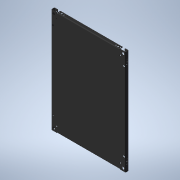
# Autodesk Inventor part: 8617.540_P1
Saved by Autodesk Inventor 2021 (Build 250183000, 183)
## iProperties
Created: 2026-08-04
Part Number: 8617.540_P1
Material: Generic
Catalog Web Link: www.3dfindit.com
Description: VX Teilmontageplatte - P1-VX Teilmontageplatte - P1
Vendor: RITTAL
Document SubType Name: Modeling
Designer: psAdmin
Manufacturer: RITTAL
Mass: 1032.29 g
Surface Area: 8360.76 cm^2
Volume: 1032.29 cm^3
Density: 1 g/cm^3
Appearance: PSOLRGB-176-176-176
Category: PARTsolutions
Company: RITTAL
Title: 8617.540_P1
Author: Cadenas PARTsolutions
Comments: VX Teilmontageplatte - P1
PSOL_IDENT_0: {$CADENAS_DATA/23d-libs/rittal/sys_zub/innenausbau/montageplatten/parts/teilmontageplatten_m51_p1.pr
PSOL_IDENT_1: j},181 {VTYP=3D},{NB=8617.540_P1},{LINA=8617.540_P1},{NN=VX Teilmontageplatte - P1},{DATE=16.02.2026
PSOL_IDENT_2: 20:13:30},{GEOMDATE=20.05.2025 11:57:00},{VERSION=},{LINEID=40},{WBVAR=},{WBNUMERIC=}  {NB=8617.540
PSOL_IDENT_3: _P1},{LINA=8617.540_P1},{KT=DUMMY},{BEST=8617.540},{INFO=PDF Katalog},{BEZ1=VX Teilmontageplatte},{B
PSOL_IDENT_4: EZ2=für neues Großschranksystem},{B=600},{BB=499},{H=800},{HH=699},{SB=600},{SH=800},{AB=600 x 800},
PSOL_IDENT_5: {VE=1},{VERS=4},{INFOPAGE=hb35_s707},{INFOPATH=hb35_s707_en.pdf},{CNSECLASS51=27-18-92-31},{CNSECLAS
PSOL_IDENT_6: S70=27-40-92-16},{CNSECLASS80=27-40-92-16},{CNSETIM40=EC000213},{BEZ3=},{DETAIL=1},{ADDGEO=1},{GEW=9
PSOL_IDENT_7: ,22},{CNSETIM80=EC000213},{CNSETIM90=EC000213},{CNSECLASS60=27-40-92-16},{UNSPSC=31-26-15-02}
NB: 8617.540_P1
NN: VX Teilmontageplatte - P1
NT: VX Teilmontageplatte - P1
NBSYN: $BEST._P1
LINA: 8617.540_P1
CATALOG: Rittal
BEST: 8617.540
INFO: PDF Katalog
BEZ1: VX Teilmontageplatte
BB: 499
HH: 699
SB: 600
SH: 800
CNSECLASS70: 27-40-92-16
CNSECLASS80: 27-40-92-16
GEW: 9,22
CNSETIM80: EC000213
CNSETIM90: EC000213
CNSECLASS60: 27-40-92-16
UNSPSC: 31-26-15-02
SUPPLIER: RITTAL
ARTICLENO: 8617.540_P1
BOMINFO: 8617.540_P1
CREATOR: CADENAS GmbH
Autodesk Inventor part; units mm, degrees
ref_plane "YZ Plane" through (0, 0, 0) normal (1, 0, 0) x (0, 1, 0)
ref_plane "XZ Plane" through (0, 0, 0) normal (0, 1, 0) x (-1, 0, 0)
ref_plane "XY Plane" through (0, 0, 0) normal (0, 0, 1) x (1, 0, 0)
sketch "Sketch_1" plane through (0, 0, 22) normal (0, 0, 1) x (1, 0, 0)
  line L0 (-244.5, 349.5) -> (-244.5, -349.5)
  line L1 (-244.5, -349.5) -> (-211.75, -349.5)
  line L2 (-211.75, -349.5) -> (-211.75, -344.5)
  arc A0 (-209.75, -344.5) -> (-211.75, -344.5) centre (-210.75, -344.5) ccw
  line L3 (-209.75, -344.5) -> (209.75, -344.5)
  arc A1 (211.75, -344.5) -> (209.75, -344.5) centre (210.75, -344.5) ccw
  line L4 (211.75, -344.5) -> (211.75, -349.5)
  line L5 (211.75, -349.5) -> (244.5, -349.5)
  line L6 (244.5, -349.5) -> (244.5, 349.5)
  line L7 (244.5, 349.5) -> (211.75, 349.5)
  line L8 (211.75, 349.5) -> (211.75, 344.5)
  arc A2 (209.75, 344.5) -> (211.75, 344.5) centre (210.75, 344.5) ccw
  line L9 (209.75, 344.5) -> (-209.75, 344.5)
  arc A3 (-211.75, 344.5) -> (-209.75, 344.5) centre (-210.75, 344.5) ccw
  line L10 (-211.75, 344.5) -> (-211.75, 349.5)
  line L11 (-211.75, 349.5) -> (-244.5, 349.5)
  circle A4 centre (237.5, 262.5) radius 6.25
  circle A5 centre (237.5, -262.5) radius 6.25
  circle A6 centre (232.5, 332.5) radius 8
  circle A7 centre (232.5, -332.5) radius 8
  circle A8 centre (213, 313) radius 4.5
  circle A9 centre (213, -313) radius 4.5
  circle A10 centre (-213, 313) radius 4.5
  circle A11 centre (-213, -313) radius 4.5
  circle A12 centre (-232.5, 332.5) radius 8
  circle A13 centre (-232.5, -332.5) radius 8
  circle A14 centre (-237.5, 262.5) radius 6.25
  circle A15 centre (-237.5, -262.5) radius 6.25
  constraints: 24 end point, 16 centre point, 8 point on circle
extrude "Extrusion1" add sketch "Sketch_1" against normal blind 2.5
sketch "Sketch_2" plane through (0, 0, 0) normal (0, 1, 0) x (1, 0, 0)
  line L0 (244.5, -19.5) -> (244.5, -22)
  arc A0 (244.5, -22) -> (249.5, -17) centre (244.5, -17) ccw
  line L1 (249.5, -17) -> (247, -17)
  arc A1 (244.5, -19.5) -> (247, -17) centre (244.5, -17) ccw
  constraints: 4 end point, 4 point on circle, 2 centre point
extrude "Extrusion2" add sketch "Sketch_2" along normal mid plane 699
sketch "Sketch_3" plane through (0, 0, 0) normal (0, 1, 0) x (1, 0, 0)
  arc A0 (-249.5, -17) -> (-244.5, -22) centre (-244.5, -17) ccw
  line L0 (-244.5, -22) -> (-244.5, -19.5)
  arc A1 (-247, -17) -> (-244.5, -19.5) centre (-244.5, -17) ccw
  line L1 (-247, -17) -> (-249.5, -17)
  constraints: 4 end point, 4 point on circle, 2 centre point
extrude "Extrusion3" add sketch "Sketch_3" along normal mid plane 699
sketch "Sketch_4" plane through (249.5, 0, 0) normal (1, 0, 0) x (0, 0, -1)
  line L0 (-17, 349.5) -> (-17, -349.5)
  line L1 (-17, -349.5) -> (-5, -349.5)
  line L2 (-5, -349.5) -> (-5, 349.5)
  line L3 (-5, 349.5) -> (-17, 349.5)
  circle A0 centre (-11, 304.5) radius 3.5
  circle A1 centre (-11, 274.5) radius 3.5
  circle A2 centre (-11, -304.5) radius 3.5
  circle A3 centre (-11, -274.5) radius 3.5
  circle A4 centre (-11, 289.5) radius 5.5
  circle A5 centre (-11, -289.5) radius 5.5
  constraints: 8 end point, 6 centre point
extrude "Extrusion4" add sketch "Sketch_4" against normal blind 2.5
sketch "Sketch_5" plane through (-249.5, 0, 0) normal (1, 0, 0) x (0, 0, -1)
  line L0 (-17, 349.5) -> (-17, -349.5)
  line L1 (-17, -349.5) -> (-5, -349.5)
  line L2 (-5, -349.5) -> (-5, 349.5)
  line L3 (-5, 349.5) -> (-17, 349.5)
  circle A0 centre (-11, 304.5) radius 3.5
  circle A1 centre (-11, 274.5) radius 3.5
  circle A2 centre (-11, -304.5) radius 3.5
  circle A3 centre (-11, -274.5) radius 3.5
  circle A4 centre (-11, 289.5) radius 5.5
  circle A5 centre (-11, -289.5) radius 5.5
  constraints: 8 end point, 6 centre point
extrude "Extrusion5" add sketch "Sketch_5" along normal blind 2.5
sketch "Sketch_6" plane through (0, 0, 0) normal (0, 1, 0) x (1, 0, 0)
  arc A0 (247, -5) -> (244.5, -2.5) centre (244.5, -5) ccw
  line L0 (247, -5) -> (249.5, -5)
  arc A1 (249.5, -5) -> (244.5, 0) centre (244.5, -5) ccw
  line L1 (244.5, 0) -> (244.5, -2.5)
  constraints: 4 end point, 4 point on circle, 2 centre point
extrude "Extrusion6" add sketch "Sketch_6" along normal mid plane 699
sketch "Sketch_7" plane through (0, 0, 0) normal (0, 1, 0) x (1, 0, 0)
  line L0 (-249.5, -5) -> (-247, -5)
  arc A0 (-244.5, -2.5) -> (-247, -5) centre (-244.5, -5) ccw
  line L1 (-244.5, -2.5) -> (-244.5, 0)
  arc A1 (-244.5, 0) -> (-249.5, -5) centre (-244.5, -5) ccw
  constraints: 4 end point, 4 point on circle, 2 centre point
extrude "Extrusion7" add sketch "Sketch_7" along normal mid plane 699
sketch "Sketch_8" plane through (0, 0, 0) normal (0, 0, 1) x (1, 0, 0)
  arc A0 (225, -347) -> (227.5, -349.5) centre (227.5, -347) ccw
  line L0 (227.5, -349.5) -> (244.5, -349.5)
  line L1 (244.5, -349.5) -> (244.5, 349.5)
  line L2 (244.5, 349.5) -> (227.5, 349.5)
  arc A1 (227.5, 349.5) -> (225, 347) centre (227.5, 347) ccw
  line L3 (225, 347) -> (225, 331)
  arc A2 (225, 331) -> (226, 330) centre (226, 331) ccw
  line L4 (226, 330) -> (227.3, 330)
  arc A3 (227.3, 330) -> (228.3, 331) centre (227.3, 331) ccw
  line L5 (228.3, 331) -> (228.3, 332.5)
  arc A4 (236.7, 332.5) -> (228.3, 332.5) centre (232.5, 332.5) ccw
  line L6 (236.7, 332.5) -> (236.7, 330)
  line L7 (236.7, 330) -> (239.1825, 325.1277)
  arc A5 (240, 321.7228) -> (239.1825, 325.1277) centre (232.5, 321.7228) ccw
  line L8 (240, 321.7228) -> (240, 315.5)
  line L9 (240, 315.5) -> (227.5, 315.5)
  arc A6 (227.5, 315.5) -> (225, 313) centre (227.5, 313) ccw
  line L10 (225, 313) -> (225, -313)
  arc A7 (225, -313) -> (227.5, -315.5) centre (227.5, -313) ccw
  line L11 (227.5, -315.5) -> (240, -315.5)
  line L12 (240, -315.5) -> (240, -321.7228)
  arc A8 (239.1825, -325.1277) -> (240, -321.7228) centre (232.5, -321.7228) ccw
  line L13 (239.1825, -325.1277) -> (236.7, -330)
  line L14 (236.7, -330) -> (236.7, -332.5)
  arc A9 (228.3, -332.5) -> (236.7, -332.5) centre (232.5, -332.5) ccw
  line L15 (228.3, -332.5) -> (228.3, -331)
  arc A10 (228.3, -331) -> (227.3, -330) centre (227.3, -331) ccw
  line L16 (227.3, -330) -> (226, -330)
  arc A11 (226, -330) -> (225, -331) centre (226, -331) ccw
  line L17 (225, -331) -> (225, -347)
  circle A12 centre (237.5, 302) radius 3.5
  circle A13 centre (237.5, 262.5) radius 3.5
  circle A14 centre (237.5, -302) radius 3.5
  circle A15 centre (237.5, -262.5) radius 3.5
  constraints: 36 end point, 24 point on circle, 16 centre point
extrude "Extrusion8" add sketch "Sketch_8" along normal blind 2.5
sketch "Sketch_9" plane through (0, 0, 0) normal (0, 0, 1) x (1, 0, 0)
  line L0 (-244.5, -349.5) -> (-227.5, -349.5)
  arc A0 (-227.5, -349.5) -> (-225, -347) centre (-227.5, -347) ccw
  line L1 (-225, -347) -> (-225, -331)
  arc A1 (-225, -331) -> (-226, -330) centre (-226, -331) ccw
  line L2 (-226, -330) -> (-227.3, -330)
  arc A2 (-227.3, -330) -> (-228.3, -331) centre (-227.3, -331) ccw
  line L3 (-228.3, -331) -> (-228.3, -332.5)
  arc A3 (-236.7, -332.5) -> (-228.3, -332.5) centre (-232.5, -332.5) ccw
  line L4 (-236.7, -332.5) -> (-236.7, -330)
  line L5 (-236.7, -330) -> (-239.1825, -325.1277)
  arc A4 (-240, -321.7228) -> (-239.1825, -325.1277) centre (-232.5, -321.7228) ccw
  line L6 (-240, -321.7228) -> (-240, -315.5)
  line L7 (-240, -315.5) -> (-227.5, -315.5)
  arc A5 (-227.5, -315.5) -> (-225, -313) centre (-227.5, -313) ccw
  line L8 (-225, -313) -> (-225, 313)
  arc A6 (-225, 313) -> (-227.5, 315.5) centre (-227.5, 313) ccw
  line L9 (-227.5, 315.5) -> (-240, 315.5)
  line L10 (-240, 315.5) -> (-240, 321.7228)
  arc A7 (-239.1825, 325.1277) -> (-240, 321.7228) centre (-232.5, 321.7228) ccw
  line L11 (-239.1825, 325.1277) -> (-236.7, 330)
  line L12 (-236.7, 330) -> (-236.7, 332.5)
  arc A8 (-228.3, 332.5) -> (-236.7, 332.5) centre (-232.5, 332.5) ccw
  line L13 (-228.3, 332.5) -> (-228.3, 331)
  arc A9 (-228.3, 331) -> (-227.3, 330) centre (-227.3, 331) ccw
  line L14 (-227.3, 330) -> (-226, 330)
  arc A10 (-226, 330) -> (-225, 331) centre (-226, 331) ccw
  line L15 (-225, 331) -> (-225, 347)
  arc A11 (-225, 347) -> (-227.5, 349.5) centre (-227.5, 347) ccw
  line L16 (-227.5, 349.5) -> (-244.5, 349.5)
  line L17 (-244.5, 349.5) -> (-244.5, -349.5)
  circle A12 centre (-237.5, 302) radius 3.5
  circle A13 centre (-237.5, 262.5) radius 3.5
  circle A14 centre (-237.5, -302) radius 3.5
  circle A15 centre (-237.5, -262.5) radius 3.5
  constraints: 36 end point, 24 point on circle, 16 centre point
extrude "Extrusion9" add sketch "Sketch_9" along normal blind 2.5
sketch "Sketch_10" plane through (0, 0, 0) normal (1, 0, 0) x (0, 0, -1)
  line L0 (-22, 344.5) -> (-19.5, 344.5)
  arc A0 (-17, 347) -> (-19.5, 344.5) centre (-17, 344.5) ccw
  line L1 (-17, 347) -> (-17, 349.5)
  arc A1 (-17, 349.5) -> (-22, 344.5) centre (-17, 344.5) ccw
  constraints: 4 end point, 4 point on circle, 2 centre point
extrude "Extrusion10" add sketch "Sketch_10" along normal mid plane 419.5
sketch "Sketch_11" plane through (0, 0, 0) normal (1, 0, 0) x (0, 0, -1)
  arc A0 (-22, -344.5) -> (-17, -349.5) centre (-17, -344.5) ccw
  line L0 (-17, -349.5) -> (-17, -347)
  arc A1 (-19.5, -344.5) -> (-17, -347) centre (-17, -344.5) ccw
  line L1 (-19.5, -344.5) -> (-22, -344.5)
  constraints: 4 end point, 4 point on circle, 2 centre point
extrude "Extrusion11" add sketch "Sketch_11" along normal mid plane 419.5
sketch "Sketch_12" plane through (0, 349.5, 0) normal (0, 1, 0) x (1, 0, 0)
  line L0 (-209.75, -2.5) -> (-209.75, -17)
  line L1 (-209.75, -17) -> (209.75, -17)
  line L2 (209.75, -17) -> (209.75, -2.5)
  arc A0 (209.75, -2.5) -> (207.25, 0) centre (207.25, -2.5) ccw
  line L3 (207.25, 0) -> (-207.25, 0)
  arc A1 (-207.25, 0) -> (-209.75, -2.5) centre (-207.25, -2.5) ccw
  circle A2 centre (204.5, -11) radius 4
  circle A3 centre (189.5, -11) radius 5.5
  circle A4 centre (174.5, -11) radius 4
  circle A5 centre (-174.5, -11) radius 4
  circle A6 centre (-189.5, -11) radius 5.5
  circle A7 centre (-204.5, -11) radius 4
  constraints: 8 centre point, 8 end point, 4 point on circle
extrude "Extrusion12" add sketch "Sketch_12" against normal blind 2.5
sketch "Sketch_13" plane through (0, -349.5, 0) normal (0, 1, 0) x (1, 0, 0)
  line L0 (-209.75, -2.5) -> (-209.75, -17)
  line L1 (-209.75, -17) -> (209.75, -17)
  line L2 (209.75, -17) -> (209.75, -2.5)
  arc A0 (209.75, -2.5) -> (207.25, 0) centre (207.25, -2.5) ccw
  line L3 (207.25, 0) -> (-207.25, 0)
  arc A1 (-207.25, 0) -> (-209.75, -2.5) centre (-207.25, -2.5) ccw
  circle A2 centre (204.5, -11) radius 4
  circle A3 centre (189.5, -11) radius 5.5
  circle A4 centre (174.5, -11) radius 4
  circle A5 centre (-174.5, -11) radius 4
  circle A6 centre (-189.5, -11) radius 5.5
  circle A7 centre (-204.5, -11) radius 4
  constraints: 8 centre point, 8 end point, 4 point on circle
extrude "Extrusion13" add sketch "Sketch_13" along normal blind 2.5
ref_plane "P1_XY" through (0, 0, 0) normal (0, 0, 1) x (1, 0, 0)
ref_plane "P1_YZ" through (0, 0, 0) normal (1, 0, 0) x (0, 1, 0)
ref_plane "P1_ZX" through (0, 0, 0) normal (0, 1, 0) x (0, 0, 1)
ref_plane "P21_XY" through (232.5, 332.5, -1) normal (0, 0, 1) x (1, 0, 0)
ref_plane "P21_YZ" through (232.5, 332.5, -1) normal (1, 0, 0) x (0, 1, 0)
ref_plane "P21_ZX" through (232.5, 332.5, -1) normal (0, 1, 0) x (0, 0, 1)
ref_plane "P22_XY" through (-232.5, 332.5, -1) normal (0, 0, 1) x (1, 0, 0)
ref_plane "P22_YZ" through (-232.5, 332.5, -1) normal (1, 0, 0) x (0, 1, 0)
ref_plane "P22_ZX" through (-232.5, 332.5, -1) normal (0, 1, 0) x (0, 0, 1)
ref_plane "P23_XY" through (232.5, -332.5, -1) normal (0, 0, 1) x (1, 0, 0)
ref_plane "P23_YZ" through (232.5, -332.5, -1) normal (1, 0, 0) x (0, 1, 0)
ref_plane "P23_ZX" through (232.5, -332.5, -1) normal (0, 1, 0) x (0, 0, 1)
ref_plane "P24_XY" through (-232.5, -332.5, -1) normal (0, 0, 1) x (1, 0, 0)
ref_plane "P24_YZ" through (-232.5, -332.5, -1) normal (1, 0, 0) x (0, 1, 0)
ref_plane "P24_ZX" through (-232.5, -332.5, -1) normal (0, 1, 0) x (0, 0, 1)
ref_plane "P31_XY" through (232.5, 332.5, 0) normal (0, 0, 1) x (1, 0, 0)
ref_plane "P31_YZ" through (232.5, 332.5, 0) normal (1, 0, 0) x (0, 1, 0)
ref_plane "P31_ZX" through (232.5, 332.5, 0) normal (0, 1, 0) x (0, 0, 1)
ref_plane "P32_XY" through (-232.5, 332.5, 0) normal (0, 0, 1) x (1, 0, 0)
ref_plane "P32_YZ" through (-232.5, 332.5, 0) normal (1, 0, 0) x (0, 1, 0)
ref_plane "P32_ZX" through (-232.5, 332.5, 0) normal (0, 1, 0) x (0, 0, 1)
ref_plane "P33_XY" through (232.5, -332.5, 0) normal (0, 0, 1) x (1, 0, 0)
ref_plane "P33_YZ" through (232.5, -332.5, 0) normal (1, 0, 0) x (0, 1, 0)
ref_plane "P33_ZX" through (232.5, -332.5, 0) normal (0, 1, 0) x (0, 0, 1)
ref_plane "P34_XY" through (-232.5, -332.5, 0) normal (0, 0, 1) x (1, 0, 0)
ref_plane "P34_YZ" through (-232.5, -332.5, 0) normal (1, 0, 0) x (0, 1, 0)
ref_plane "P34_ZX" through (-232.5, -332.5, 0) normal (0, 1, 0) x (0, 0, 1)
body "Solid1"
